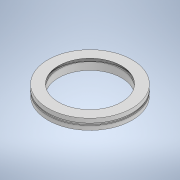
# Autodesk Inventor part: Маслосъемное кольцо
Saved by Autodesk Inventor 2021 (Build 250183000, 183)
## iProperties
Created: 2020-11-17
Part Number: Маслосъемное кольцо
Material: Типовые
Document SubType Name: Modeling
Designer: Тимоха
Density: 1 g/cm^3
Appearance: По умолчанию
Author: Тимоха
Autodesk Inventor part; units mm, degrees
ref_plane "YZ Plane" through (0, 0, 0) normal (1, 0, 0) x (0, 1, 0)
ref_plane "XZ Plane" through (0, 0, 0) normal (0, 1, 0) x (-1, 0, 0)
ref_plane "XY Plane" through (0, 0, 0) normal (0, 0, 1) x (1, 0, 0)
sketch "Эскиз1" plane through (0, 0, 0) normal (0, 0, 1) x (1, 0, 0)
  line L0 (0, 0) -> (30, 0)
  line L1 (30, 0) -> (40, 0)
  line L2 (40, -10) -> (30, -10)
  line L3 (30, -10) -> (30, -2.8868)
  line L4 (30, 0) -> (35.1962, -3)
  line L5 (33.9462, -5.1651) -> (30, -2.8868)
  arc A0 (33.9462, -5.1651) -> (35.1962, -3) centre (34.5712, -4.0825) ccw
  arc A1 (39, -4) -> (39, -6) centre (39, -5) ccw
  line L6 (39, -6) -> (40, -6)
  line L7 (39, -4) -> (40, -4)
  line L8 (40, 0) -> (40, -4)
  line L9 (40, -6) -> (40, -10)
  line L10 (0, -12) -> (0, 2) projected
  dimension "d0" = 30
  dimension "d1" = 10
  dimension "d2" = 10
  dimension "d3" = 6
  dimension "d5" = 30
  dimension "d7" = 2
  constraints: 20 end point, 9 perpendicular, 4 point on circle, 2 centre point, 2 horizontal, 2 tangent
  measures "d0" distance of L0.start L0.end
  measures "d1" distance of L0.end L1.end
  measures "d2" distance of L1.end L2.start
  measures "d3" distance of L0.end L4.end
  measures "d5" angle of L1 L4
  measures "d7" diameter of A1
revolve "Вращение1" add sketch "Эскиз1" angle 360 about axis through (0, -10, 0) along (0, 1, 0)
